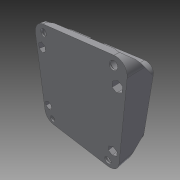
# Autodesk Inventor part: bottom
Saved by Autodesk Inventor 2014 (Build 180170000, 170)
## iProperties
Created: 2016-03-14
Part Number: bottom
Material: Generic
Document SubType Name: Modeling
Designer: buben
Density: 1 g/cm^3
Appearance: Default
Author: buben
Autodesk Inventor part; units mm, degrees
ref_plane "YZ Plane" through (0, 0, 0) normal (1, 0, 0) x (0, 1, 0)
ref_plane "XZ Plane" through (0, 0, 0) normal (0, 1, 0) x (-1, 0, 0)
ref_plane "XY Plane" through (0, 0, 0) normal (0, 0, 1) x (1, 0, 0)
sketch "Sketch1" plane through (0, 0, 0) normal (0, 1, 0) x (-1, 0, 0)
  line L0 (-3, -49.5) -> (-49.5, -49.5) construction
  line L1 (-49.5, -49.5) -> (-49.5, -3) construction
  line L2 (-49.5, -3) -> (-3, -3) construction
  line L3 (-3, -3) -> (-3, -49.5) construction
  line L4 (0, 0) -> (-52.5, 0)
  line L5 (-52.5, 0) -> (-52.5, -52.5)
  line L6 (-52.5, -52.5) -> (0, -52.5)
  line L7 (0, -52.5) -> (0, 0)
  point P0 (-3, -26.25)
  point P1 (0, -26.25)
  point P2 (-26.25, -3)
  point P3 (-26.25, 0)
  dimension "d0" = 46.5
  dimension "d1" = 46.5
  dimension "d2" = 52.5
  dimension "d3" = 52.5
  constraints: 16 end point, 4 midpoint, 4 parallel, 2 horizontal, 2 perpendicular, 1 horizontal alignment, 1 vertical alignment
  measures "d0" distance of L1.end L2.end
  measures "d1" distance of L0.end L1.end
  measures "d2" distance of L4.start L4.end
  measures "d3" distance of L6.end L4.start
extrude "Extrusion1" add sketch "Sketch1" along normal blind 3
sketch "Sketch2" plane through (0, 3, 0) normal (0, 1, 0) x (1, 0, 0)
  line L0 (0, 0) -> (52.5, 0) projected
  line L1 (0, 52.5) -> (0, 0) projected
  line L2 (0, 52.5) -> (52.5, 52.5)
  line L3 (52.5, 52.5) -> (52.5, 0)
  line L4 (52.5, 0) -> (0, 0)
  line L5 (0, 0) -> (0, 52.5)
  line L6 (3, 49.5) -> (49.5, 49.5)
  line L7 (49.5, 49.5) -> (49.5, 3)
  line L8 (49.5, 3) -> (3, 3)
  line L9 (3, 3) -> (3, 49.5)
  point P0 (3, 26.25)
  point P1 (0, 26.25)
  point P2 (26.25, 3)
  point P3 (26.25, 0)
  dimension "d6" = 3
  dimension "d7" = 3
  constraints: 16 end point, 4 midpoint, 4 parallel, 2 horizontal, 2 perpendicular, 1 horizontal alignment, 1 vertical alignment
  measures "d6" distance between parallel lines of L5 L9
  measures "d7" distance between parallel lines of L0 L8
extrude "Extrusion2" add sketch "Sketch2" along normal blind 18.5
sketch "Sketch3" plane through (0, 21.5, 0) normal (0, 1, 0) x (1, 0, 0)
  line L0 (49.5, 3) -> (3, 3) projected
  line L1 (3, 3) -> (3, 49.5) projected
  line L2 (3, 49.5) -> (49.5, 49.5) projected
  line L3 (52.5, 52.5) -> (0, 52.5) projected
  line L4 (0, 0) -> (52.5, 0) projected
  line L5 (16.69, 3) -> (26.69, 3)
  line L6 (26.69, 3) -> (26.69, 0)
  line L7 (26.69, 0) -> (16.69, 0)
  line L8 (16.69, 0) -> (16.69, 3)
  line L9 (3.39, 49.11) -> (49.11, 49.11) construction
  line L10 (49.11, 49.11) -> (49.11, 3.39) construction
  line L11 (49.11, 3.39) -> (3.39, 3.39) construction
  line L12 (3.39, 3.39) -> (3.39, 49.11) construction
  line L13 (32.96, 52.5) -> (46.46, 52.5)
  line L14 (46.46, 52.5) -> (46.46, 49.5)
  line L15 (46.46, 49.5) -> (32.96, 49.5)
  line L16 (32.96, 49.5) -> (32.96, 52.5)
  point P0 (3.39, 26.25)
  point P1 (3, 26.25)
  point P2 (26.25, 3.39)
  point P3 (26.25, 0)
  point P4 (21.69, 0)
  point P5 (39.71, 52.5)
  dimension "d10" = 10
  dimension "d11" = 45.72
  dimension "d12" = 18.3
  dimension "d13" = 13.5
  dimension "d14" = 9.4
  constraints: 24 end point, 6 midpoint, 6 parallel, 4 perpendicular, 4 point on line, 3 horizontal, 1 horizontal alignment, 1 vertical alignment
  measures "d10" distance between parallel lines of L6 L8
  measures "d11" distance of L10.end L11.end
  measures "d12" horizontal distance of L11.end point (21.69, 0)
  measures "d13" distance of L13.start L13.end
  measures "d14" horizontal distance of L9.end point (39.71, 52.5)
extrude "Extrusion3" cut sketch "Sketch3" against normal blind 12.4
sketch "Sketch4" plane through (0, 3, 0) normal (0, 1, 0) x (1, 0, 0)
  line L0 (49.5, 49.5) -> (3, 49.5) projected
  line L1 (3, 49.5) -> (3, 3) projected
  circle A0 centre (5.93, 21.89) radius 2
  circle A1 centre (30.59, 46.57) radius 2
  circle A2 centre (39.11, 5.93) radius 2
  circle A3 centre (46.57, 30.81) radius 2
  line L2 (49.11, 3.39) -> (3.39, 3.39) construction
  line L3 (3.39, 3.39) -> (3.39, 49.11) construction
  line L4 (3.39, 49.11) -> (49.11, 49.11) construction
  line L5 (49.11, 49.11) -> (49.11, 3.39) construction
  point P0 (0, 0)
  point P1 (26.25, 49.11)
  point P2 (26.25, 49.5)
  point P3 (3.39, 26.25)
  point P4 (3, 26.25)
  dimension "d17" = 4
  dimension "d18" = 45.72
  dimension "d19" = 2.54
  dimension "d20" = 18.5
  dimension "d21" = 2.54
  dimension "d23" = 2.54
  dimension "d25" = 2.54
  dimension "d26" = 27.2
  dimension "d86" = 10
  dimension "d87" = 18.3
  constraints: 8 end point, 4 centre point, 4 midpoint, 3 equal radius, 2 parallel, 2 perpendicular, 1 horizontal, 1 horizontal alignment, 1 vertical alignment
  measures "d17" diameter of A0
  measures "d18" distance of L2.end L3.end
  measures "d19" distance from line of L3 A0.centre
  measures "d20" distance from line of L2 A0.centre
  measures "d21" distance from line of L2 A2.centre
  measures "d23" distance from line of L5 A3.centre
  measures "d25" distance from line of L4 A1.centre
  measures "d26" distance from line of L3 A1.centre
  measures "d86" distance from line of L5 A2.centre
  measures "d87" distance from line of L4 A3.centre
extrude "Extrusion4" add sketch "Sketch4" along normal blind 5
sketch "Sketch5" plane through (0, 21.5, 0) normal (0, 1, 0) x (1, 0, 0)
  line L0 (3, 3) -> (3, 49.5) projected
  line L1 (26.69, 3) -> (26.69, 0) projected
  line L2 (26.69, 0) -> (52.5, 0) projected
  line L3 (52.5, 0) -> (52.5, 52.5) projected
  line L4 (52.5, 52.5) -> (46.46, 52.5) projected
  line L5 (46.46, 52.5) -> (46.46, 49.5) projected
  line L6 (46.46, 49.5) -> (49.5, 49.5) projected
  line L7 (49.5, 49.5) -> (49.5, 3) projected
  line L8 (49.5, 3) -> (26.69, 3) projected
  line L9 (0, 52.5) -> (-7, 52.5)
  line L10 (-7, 52.5) -> (-7, 0)
  line L11 (-7, 0) -> (0, 0)
  line L12 (0, 0) -> (0, 52.5)
  line L13 (52.5, 52.5) -> (59.5, 52.5)
  line L14 (59.5, 52.5) -> (59.5, 0)
  line L15 (59.5, 0) -> (52.5, 0)
  line L16 (52.5, 0) -> (52.5, 52.5)
  dimension "d29" = 10
  dimension "d30" = 10
  constraints: 16 end point, 4 parallel, 2 horizontal, 2 perpendicular
  measures "d29" distance between parallel lines of L10 L0
  measures "d30" distance between parallel lines of L7 L14
extrude "Extrusion5" add sketch "Sketch5" against normal up to surface (21.5 mm away) contours L3 L13 L14 L15 | L12 L11 L10 L9
sketch "Sketch6" plane through (0, 21.5, 0) normal (0, 1, 0) x (1, 0, 0)
  line L0 (3, 3) -> (3, 49.5) projected
  line L1 (32.96, 52.5) -> (-7, 52.5) projected
  line L2 (-7, 52.5) -> (-7, 0) projected
  line L3 (-7, 0) -> (16.69, 0) projected
  line L4 (26.69, 3) -> (26.69, 0) projected
  line L5 (26.69, 0) -> (59.5, 0) projected
  line L6 (59.5, 0) -> (59.5, 52.5) projected
  line L7 (59.5, 52.5) -> (46.46, 52.5) projected
  line L8 (46.46, 52.5) -> (46.46, 49.5) projected
  line L9 (46.46, 49.5) -> (49.5, 49.5) projected
  line L10 (49.5, 49.5) -> (49.5, 3) projected
  line L11 (49.5, 3) -> (26.69, 3) projected
  line L12 (54.5, 5) -> (-2, 5) construction
  line L13 (-2, 5) -> (-2, 47.5) construction
  line L14 (-2, 47.5) -> (54.5, 47.5) construction
  line L15 (54.5, 47.5) -> (54.5, 5) construction
  point P0 (0, 0)
  dimension "d33" = 10
  dimension "d34" = 5
  dimension "d35" = 5
  dimension "d37" = 5
  dimension "d38" = 5
  constraints: 8 end point, 4 coincident, 2 parallel, 1 horizontal, 1 perpendicular
  measures "d33" distance between parallel lines of L2 L0
  measures "d34" distance between parallel lines of L2 L13
  measures "d35" distance between parallel lines of L6 L15
  measures "d37" distance between parallel lines of L3 L12
  measures "d38" distance between parallel lines of L1 L14
hole "Hole1" at (-2, 21.5, -47.5) at (54.5, 21.5, -47.5) at (54.5, 21.5, -5) at (-2, 21.5, -5) direction (0, -1, 0) diameter 3 end through all
sketch "Sketch7" plane through (59.5, 21.5, 0) normal (1, 0, 0) x (0, 0, -1)
  line L0 (0, -21.5) -> (-10, -21.5)
  line L1 (-10, -21.5) -> (-10, -16.5)
  line L2 (-10, -16.5) -> (0, -16.5)
  line L3 (0, -16.5) -> (0, -21.5)
  line L4 (52.5, -21.5) -> (62.5, -21.5)
  line L5 (62.5, -21.5) -> (62.5, -16.5)
  line L6 (62.5, -16.5) -> (52.5, -16.5)
  line L7 (52.5, -16.5) -> (52.5, -21.5)
  dimension "d46" = 5
  dimension "d47" = 10
  constraints: 16 end point, 4 parallel, 2 equal length, 2 horizontal, 2 perpendicular
  measures "d46" distance of L0.end L1.end
  measures "d47" distance of L0.start L0.end
extrude "Extrusion6" add sketch "Sketch7" against normal up to surface (66.5 mm away)
chamfer "Chamfer1" distance 10 angle 45 2 edges at (26.25, 5, 0) (26.25, 5, -52.5)
sketch "Sketch9" plane through (0, 21.5, 0) normal (0, 1, 0) x (1, 0, 0)
  line L0 (32.96, 52.5) -> (-7, 52.5) projected
  line L1 (-7, 52.5) -> (-7, 0) projected
  line L2 (-7, 0) -> (16.69, 0) projected
  circle A0 centre (54.5, 5) radius 1.5 projected
  circle A1 centre (54.5, 47.5) radius 1.5 projected
  line L3 (26.69, 3) -> (26.69, 0) projected
  line L4 (26.69, 0) -> (59.5, 0) projected
  line L5 (59.5, 0) -> (59.5, 52.5) projected
  line L6 (59.5, 52.5) -> (46.46, 52.5) projected
  line L7 (46.46, 52.5) -> (46.46, 49.5) projected
  line L8 (46.46, 49.5) -> (49.5, 49.5) projected
  line L9 (49.5, 49.5) -> (49.5, 3) projected
  line L10 (49.5, 3) -> (26.69, 3) projected
  line L11 (1, 57.5) -> (51.5, 57.5) construction
  line L12 (51.5, 57.5) -> (51.5, -5) construction
  line L13 (51.5, -5) -> (1, -5) construction
  line L14 (1, -5) -> (1, 57.5) construction
  circle A2 centre (1, 57.5) radius 4.5
  circle A3 centre (51.5, 57.5) radius 4.5
  circle A4 centre (51.5, -5) radius 4.5
  circle A5 centre (1, -5) radius 4.5
  point P0 (0, 0)
  dimension "d54" = 9
  dimension "d55" = 8
  dimension "d57" = 8
  dimension "d58" = 5
  dimension "d59" = 5
  constraints: 8 end point, 4 centre point, 4 coincident, 3 equal radius, 2 parallel, 1 horizontal, 1 perpendicular
  measures "d54" diameter of A2
  measures "d55" distance between parallel lines of L1 L14
  measures "d57" distance between parallel lines of L12 L5
  measures "d58" distance between parallel lines of L0 L11
  measures "d59" distance between parallel lines of L2 L13
extrude "Extrusion7" cut sketch "Sketch9" against normal up to surface (18.5 mm away) contours A2 | A3 | A4 | A5
sketch "Sketch10" plane through (1, 3, -57.5) normal (0, 1, 0) x (1, 0, 0)
  circle A0 centre (0, 0) radius 4.5 projected
  circle A1 centre (50.5, 0) radius 4.5 projected
  circle A2 centre (0, -62.5) radius 4.5 projected
  circle A3 centre (50.5, -62.5) radius 4.5 projected
  point P0 (0, 5)
  point P1 (-1, -57.5)
  constraints: 1 vertical alignment
hole "Hole2" at (1, 3, -57.5) at (51.5, 3, -57.5) at (1, 3, 5) at (51.5, 3, 5) direction (0, -1, 0) diameter 5 end through all countersink diameter 9 countersink angle 90
sketch "Sketch11" plane through (0, 0, 0) normal (0, -1, 0) x (1, 0, 0)
  circle A0 centre (54.5, -5) radius 1.5 projected
  circle A1 centre (-2, -47.5) radius 1.5 projected
  circle A2 centre (54.5, -47.5) radius 1.5 projected
  circle A3 centre (-2, -5) radius 1.5 projected
  line L0 (-5, -6.7321) -> (-5, -3.2679)
  line L1 (-5, -3.2679) -> (-2, -1.5359)
  line L2 (-2, -1.5359) -> (1, -3.2679)
  line L3 (1, -3.2679) -> (1, -6.7321)
  line L4 (1, -6.7321) -> (-2, -8.4641)
  line L5 (-2, -8.4641) -> (-5, -6.7321)
  line L6 (-5, -49.2321) -> (-5, -45.7679)
  line L7 (-5, -45.7679) -> (-2, -44.0359)
  line L8 (-2, -44.0359) -> (1, -45.7679)
  line L9 (1, -45.7679) -> (1, -49.2321)
  line L10 (1, -49.2321) -> (-2, -50.9641)
  line L11 (-2, -50.9641) -> (-5, -49.2321)
  line L12 (57.5, -49.2321) -> (54.5, -50.9641)
  line L13 (54.5, -50.9641) -> (51.5, -49.2321)
  line L14 (51.5, -49.2321) -> (51.5, -45.7679)
  line L15 (51.5, -45.7679) -> (54.5, -44.0359)
  line L16 (54.5, -44.0359) -> (57.5, -45.7679)
  line L17 (57.5, -45.7679) -> (57.5, -49.2321)
  line L18 (57.5, -6.7321) -> (54.5, -8.4641)
  line L19 (54.5, -8.4641) -> (51.5, -6.7321)
  line L20 (51.5, -6.7321) -> (51.5, -3.2679)
  line L21 (51.5, -3.2679) -> (54.5, -1.5359)
  line L22 (54.5, -1.5359) -> (57.5, -3.2679)
  line L23 (57.5, -3.2679) -> (57.5, -6.7321)
  point P0 (0, 0)
  dimension "d72" = 6
  dimension "d73" = 6
  dimension "d74" = 6
  dimension "d75" = 6
  constraints: 48 end point, 4 coincident, 4 vertical, 52 other
  measures "d72" distance between parallel lines of L1 L4
  measures "d73" distance between parallel lines of L10 L7
  measures "d74" distance between parallel lines of L21 L18
  measures "d75" distance between parallel lines of L12 L15
extrude "Extrusion8" cut sketch "Sketch11" against normal blind 10
chamfer "Chamfer3" distance 2 angle 45 4 edges at (-3.5, 10, 5) (47, 10, 5) (47, 10, -57.5) (-3.5, 10, -57.5)
fillet "Fillet1" radius 6 4 edges at (59.5, 18.25, -52.5) (59.5, 18.25, 0) (-7, 18.25, 0) (-7, 18.25, -52.5)
fillet "Fillet2" radius 8 4 edges at (-7, 2.5, -62.5) (-7, 2.5, 10) (59.5, 2.5, 10) (59.5, 2.5, -62.5)
fillet "Fillet3" radius 4 2 edges at (16.69, 9.1, 1.45) (26.69, 9.1, 1.45)
sketch "Sketch12" plane through (0, 21.5, 0) normal (0, 1, 0) x (1, 0, 0)
  circle A0 centre (54.5, 5) radius 1.5 projected
  circle A1 centre (54.5, 47.5) radius 1.5 projected
  arc A2 (53.5, 0) -> (59.5, 6) centre (53.5, 6) ccw projected
  line L0 (59.5, 6) -> (59.5, 46.5) projected
  arc A3 (59.5, 46.5) -> (53.5, 52.5) centre (53.5, 46.5) ccw projected
  line L1 (53.5, 52.5) -> (46.46, 52.5) projected
  line L2 (46.46, 52.5) -> (46.46, 49.5) projected
  line L3 (46.46, 49.5) -> (49.5, 49.5) projected
  line L4 (49.5, 49.5) -> (49.5, 3) projected
  line L5 (49.5, 3) -> (26.69, 3) projected
  line L6 (26.69, 3) -> (26.69, 0) projected
  line L7 (26.69, 0) -> (53.5, 0) projected
  line L8 (16.69, 3) -> (26.69, 3)
  line L9 (26.69, 3) -> (26.69, 0)
  line L10 (26.69, 0) -> (16.69, 0)
  line L11 (16.69, 0) -> (16.69, 3)
  point P0 (0, 0)
  constraints: 8 end point, 2 parallel, 1 horizontal, 1 perpendicular
extrude "Extrusion9" cut sketch "Sketch12" against normal up to surface (12.4 mm away) contours L10 L11 L8 L6
equation "\"d21\" = d19"
equation "\"d23\" = d21"
equation "\"d25\" = d23"
equation "\"d30\" = d29"
equation "\"d34\" = 0.5 * d33"
equation "\"d35\" = d34"
equation "\"d38\" = d37"
equation "\"d57\" = d55"
equation "\"d59\" = d58"
equation "\"d73\" = d72"
equation "\"d74\" = d72"
equation "\"d75\" = d72"
body "Solid1"
